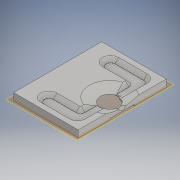
# Autodesk Inventor part: wide_access_platform_v01x
Saved by Autodesk Inventor 2016 (Build 200138000, 138)
## iProperties
Created: 2016-07-15
Part Number: wide_access_platform_v01x
Material: Generic
Document SubType Name: Modeling
Designer: stephenholtz
Density: 1 g/cm^3
Appearance: Default
Author: stephenholtz
Autodesk Inventor part; units mm, degrees
ref_plane "YZ Plane" through (0, 0, 0) normal (1, 0, 0) x (0, 1, 0)
sketch "base_rect" plane through (0, 0, 0) normal (0, 1, 0) x (-1, 0, 0)
  line L0 (-22, 30) -> (22, 30)
  line L1 (22, 30) -> (22, -30)
  line L2 (22, -30) -> (-22, -30)
  line L3 (-22, -30) -> (-22, 30)
  line L4 (-22, 30) -> (22, -30) construction
  line L5 (22, 30) -> (-22, -30) construction
  point P0 (0, 0)
  dimension "d0" = 60
  dimension "d1" = 44
  constraints: 12 end point, 2 midpoint, 2 parallel, 1 horizontal, 1 perpendicular
  measures "d0" distance of L0.end L1.end
  measures "d1" distance of L1.end L2.end
extrude "Extrusion1" add sketch "base_rect" along normal blind 4
sketch "droso_bath" plane through (0, 4, 0) normal (0, 1, 0) x (1, 0, 0)
  line L0 (-22, -30) -> (22, -30) construction
  line L1 (-22, 30) -> (-22, -30) construction
  line L2 (22, 30) -> (-22, 30) construction
  line L3 (22, -30) -> (22, 30) construction
  line L4 (-22, 0) -> (22, 0)
  line L5 (-19.5, -30) -> (-19.5, 30) construction
  circle A0 centre (-13.5, 0) radius 6
  point P0 (0, 0)
  point P1 (0, 0)
  dimension "d4" = 2.5
  dimension "d5" = 12
  constraints: 4 end point, 3 point on line, 2 midpoint, 1 centre point, 1 coincident, 1 perpendicular, 1 tangent
  measures "d4" distance between parallel lines of L5 L1
  measures "d5" diameter of A0
sketch "Sketch3" plane through (0, 4, 0) normal (0, 1, 0) x (1, 0, 0)
  line L0 (-22, 30) -> (-22, -30) construction
  line L1 (-22, -30) -> (22, -30) construction
  line L2 (22, 30) -> (-22, 30) construction
  line L3 (22, -30) -> (22, 30) construction
  line L4 (-13.5, -30) -> (-13.5, 30) construction
  circle A0 centre (-13.5, 0) radius 6 construction
  line L5 (-11.5, 0) -> (-15.5, 0) construction
  line L6 (-15.5, 0) -> (-15.5, 24)
  line L7 (-15.5, 24) -> (-11.5, 24) construction
  line L8 (-11.5, 15) -> (-11.5, 0)
  line L9 (-12.5, 24) -> (7, 24)
  line L10 (10, 21) -> (10, 21)
  line L11 (7, 18) -> (-8.5, 18)
  line L12 (-15.5, 18) -> (-15.5, 21)
  line L13 (30.8, 0) -> (-30.8, 0) construction
  arc A1 (-12.5, 24) -> (-15.5, 21) centre (-12.5, 21) ccw
  arc A2 (-8.5, 18) -> (-11.5, 15) centre (-8.5, 15) ccw
  arc A3 (7, 18) -> (10, 21) centre (7, 21) ccw
  arc A4 (10, 21) -> (7, 24) centre (7, 21) ccw
  dimension "ch_2" = 4
  dimension "d32" = 6
  dimension "d33" = 6
  dimension "d34" = 2
  dimension "d35" = 12
  dimension "d36" = 3
  constraints: 18 end point, 8 point on circle, 8 tangent, 6 point on line, 4 centre point, 4 parallel, 3 equal radius, 3 perpendicular, 2 horizontal, 1 collinear, 1 midpoint
  measures "ch_2" distance between parallel lines of L6 L8
  measures "d32" distance between parallel lines of L11 L9
  measures "d33" distance between parallel lines of L2 L9
  measures "d34" distance between parallel lines of L6 L4
  measures "d35" distance between parallel lines of L3 L10
  measures "d36" radius of A1
extrude "Extrusion2" cut sketch "droso_bath" against normal through all
chamfer "Chamfer1" distance 8 angle 20 1 edges at (-19.5, 4, 0)
extrude "Extrusion6" cut sketch "Sketch3" against normal blind 2.6 fills toward (-15.45, 19.5) open curves L12 A1 L9 A4 L10 A3 L11 A2 L8
chamfer "Chamfer3" distance 2.5 angle 45 7 edges at (-15.5, 4, -17.4282) (-14.6213, 4, -23.1213) (-2.75, 4, -24) (10, 4, -21) (-0.75, 4, -18) (-10.6213, 4, -17.1213) (-11.5, 4, -14.4282)
mirror "Mirror3" about plane through (0, 0, 0) normal (0, 0, 1) of "Extrusion6", "Chamfer3"
ref_plane "Work Plane1" through (0, 0, 8) normal (0, 0, 1) x (1, 0, 0)
sketch "Sketch7" plane through (0, 0, 0) normal (0, 0, 1) x (1, 0, 0)
  line L0 (-7.5, 0) -> (-19.5, 0) projected
  line L1 (-13.5, 1.2585) -> (-14.2266, 0)
  line L2 (22, 0) -> (-14.2266, 0)
  line L3 (-13.5, 1.2585) -> (22, 1.2585)
  line L4 (22, 1.2585) -> (22, 0)
  point P0 (0, 0)
  dimension "d67" = 60
  constraints: 8 end point, 1 collinear, 1 parallel, 1 perpendicular, 1 point on line
  measures "d67" angle of L0 L1
extrude "Extrusion9" cut sketch "Sketch7" along normal up to surface (8 mm away)
mirror "Mirror5" about plane through (0, 0, 0) normal (0, 0, 1) of "Extrusion9"
sketch "Sketch11" plane through (0, 0, 0) normal (0, -1, 0) x (1, 0, 0)
  line L0 (22, -8) -> (-14.2266, -8) construction
  line L1 (-14.2266, -8) -> (-14.2266, -5.9558) construction
  arc A0 (-14.2266, 5.9558) -> (-14.2266, -5.9558) centre (-13.5, 0) ccw construction
  line L2 (-14.2266, 5.9558) -> (-14.2266, 8) construction
  line L3 (-14.2266, 8) -> (22, 8) construction
  line L4 (22, 8) -> (22, 30) construction
  line L5 (22, 30) -> (-22, 30) construction
  line L6 (-22, 30) -> (-22, -30) construction
  line L7 (-22, -30) -> (22, -30) construction
  line L8 (22, -30) -> (22, -8) construction
  arc A1 (-13.5, -6.4678) -> (-13.5, 6.4678) centre (-13.5, 0) ccw construction
  line L9 (-13.5, -8) -> (22, -8) construction
  line L10 (22, 8) -> (22, -8) construction
  line L11 (-13.5, 8) -> (22, 8) construction
  line L12 (-22, 30) -> (-22, -30) construction
  line L13 (-14.2266, -8) -> (-22, -8) construction
  line L14 (-22, -8) -> (-22, 8) construction
  line L15 (-22, 8) -> (-14.2266, 8) construction
  line L16 (-14.2266, 8) -> (-14.2266, -8) construction
  line L17 (22, 30) -> (-22, 30)
  line L18 (-22, 30) -> (-22, 8)
  line L19 (-22, 8) -> (22, 8)
  line L20 (22, 8) -> (22, 30)
  line L21 (-22, -8) -> (22, -8)
  line L22 (22, -8) -> (22, -30)
  line L23 (22, -30) -> (-22, -30)
  line L24 (-22, -30) -> (-22, -8)
  line L25 (-13.5, -6.4678) -> (-13.5, -8) projected
  line L26 (-13.5, 6.4678) -> (-13.5, 8) projected
  point P0 (0, 0)
  constraints: 24 end point, 6 parallel, 3 horizontal, 3 perpendicular, 1 point on line
extrude "Extrusion13" add sketch "Sketch11" along normal blind 1
sketch "Sketch12" plane through (0, 1.4, 0) normal (0, 1, 0) x (1, 0, 0)
  point P0 (0, 0)
ref_plane "Work Plane2" through (-14, 4, -30) normal (-1, 0, 0) x (0, 0, 1)
sketch "Sketch13" plane through (-22, 4, -30) normal (-1, 0, 0) x (0, 0, 1)
  circle A0 centre (30, -1) radius 2.5
  line L0 (30, -4) -> (30, -1)
  dimension "d89" = 3
  dimension "d90" = 5
  constraints: 2 end point, 1 centre point, 1 coincident, 1 vertical
  measures "d89" distance of L0.start L0.end
  measures "d90" diameter of A0
sketch "Sketch14" plane through (-14, 4, -30) normal (-1, 0, 0) x (0, 0, 1)
  line L0 (38, -4) -> (22, -4) projected
  circle A0 centre (30, -1) radius 2.5 projected
  point P0 (30, -4)
  point P1 (30, -4)
loft "Loft1" cut profiles "Sketch13", "Sketch14"
ref_plane "Work Plane3" through (0, 0.2, 0) normal (0, 1, 0) x (1, 0, 0)
body "Solid1"
